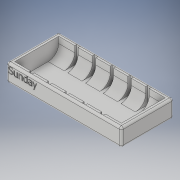
# Autodesk Inventor part: Sunday
Saved by Autodesk Inventor 2019.4 (Build 234330000, 330)
## iProperties
Created: 2020-10-20
Part Number: Sunday
Material: Generic
Document SubType Name: Modeling
Designer: daanswinters
Density: 1 g/cm^3
Appearance: Default
Author: daanswinters
Autodesk Inventor part; units mm, degrees
ref_plane "YZ Plane" through (0, 0, 0) normal (1, 0, 0) x (0, 1, 0)
ref_plane "XZ Plane" through (0, 0, 0) normal (0, 1, 0) x (-1, 0, 0)
ref_plane "XY Plane" through (0, 0, 0) normal (0, 0, 1) x (1, 0, 0)
sketch "Sketch1" plane through (0, 0, 0) normal (0, 0, 1) x (1, 0, 0)
  line L0 (55, -8.5) -> (-55, -8.5)
  line L1 (-55, -8.5) -> (-55, 8.5)
  line L2 (-55, 8.5) -> (55, 8.5)
  line L3 (55, 8.5) -> (55, -8.5)
  line L4 (55, -8.5) -> (-55, 8.5) construction
  line L5 (-55, -8.5) -> (55, 8.5) construction
  point P0 (0, 0)
  dimension "d0" = 110
  dimension "d1" = 17
  constraints: 12 end point, 2 midpoint, 2 parallel, 1 horizontal, 1 perpendicular
  measures "d0" distance of L1.end L2.end
  measures "d1" distance of L0.end L1.end
extrude "Extrusion1" add sketch "Sketch1" along normal blind 50
sketch "Sketch2" plane through (-55, 8.5, 0) normal (0, 1, 0) x (1, 0, 0)
  line L0 (0, 0) -> (0, -50) projected
  line L1 (110, -50) -> (0, -50)
  line L2 (0, -50) -> (0, 0)
  line L3 (0, 0) -> (110, 0)
  line L4 (110, 0) -> (110, -50)
  line L5 (110, -50) -> (0, 0) construction
  line L6 (0, -50) -> (110, 0) construction
  line L7 (106, -46) -> (106, -4)
  line L8 (4, -4) -> (4, -46)
  line L9 (56.15, -2) -> (53.85, -2)
  line L10 (53.85, -48) -> (56.15, -48)
  line L11 (56.15, -2) -> (53.85, -48) construction
  line L12 (53.85, -2) -> (56.15, -48) construction
  line L13 (73.15, -2) -> (70.85, -2)
  line L14 (70.85, -48) -> (73.15, -48)
  line L15 (73.15, -2) -> (70.85, -48) construction
  line L16 (70.85, -2) -> (73.15, -48) construction
  line L17 (0, -25) -> (110, -25) construction
  line L18 (87.85, -2) -> (90.15, -2)
  line L19 (90.15, -48) -> (87.85, -48)
  line L20 (87.85, -2) -> (90.15, -48) construction
  line L21 (90.15, -2) -> (87.85, -48) construction
  line L22 (36.85, -2) -> (39.15, -2)
  line L23 (39.15, -48) -> (36.85, -48)
  line L24 (36.85, -2) -> (39.15, -48) construction
  line L25 (39.15, -2) -> (36.85, -48) construction
  line L26 (19.85, -2) -> (22.15, -2)
  line L27 (22.15, -48) -> (19.85, -48)
  line L28 (19.85, -2) -> (22.15, -48) construction
  line L29 (22.15, -2) -> (19.85, -48) construction
  line L30 (90.15, -2) -> (90.15, -4)
  line L31 (90.15, -46) -> (90.15, -48)
  line L32 (87.85, -48) -> (87.85, -46)
  line L33 (87.85, -4) -> (87.85, -2)
  line L34 (73.15, -48) -> (73.15, -46)
  line L35 (73.15, -4) -> (73.15, -2)
  line L36 (70.85, -2) -> (70.85, -4)
  line L37 (70.85, -46) -> (70.85, -48)
  line L38 (56.15, -4) -> (56.15, -2)
  line L39 (53.85, -2) -> (53.85, -4)
  line L40 (53.85, -46) -> (53.85, -48)
  line L41 (56.15, -48) -> (56.15, -46)
  line L42 (39.15, -2) -> (39.15, -4)
  line L43 (39.15, -46) -> (39.15, -48)
  line L44 (36.85, -48) -> (36.85, -46)
  line L45 (36.85, -4) -> (36.85, -2)
  line L46 (22.15, -2) -> (22.15, -4)
  line L47 (19.85, -48) -> (19.85, -46)
  line L48 (19.85, -4) -> (19.85, -2)
  line L49 (22.15, -46) -> (22.15, -48)
  line L50 (4, -46) -> (19.95, -46)
  line L51 (22.05, -46) -> (36.95, -46)
  line L52 (39.05, -46) -> (53.95, -46)
  line L53 (56.05, -46) -> (70.95, -46)
  line L54 (73.05, -46) -> (87.95, -46)
  line L55 (90.05, -46) -> (106, -46)
  line L56 (106, -4) -> (90.05, -4)
  line L57 (87.95, -4) -> (73.05, -4)
  line L58 (70.95, -4) -> (56.05, -4)
  line L59 (53.95, -4) -> (39.05, -4)
  line L60 (36.95, -4) -> (22.05, -4)
  line L61 (19.95, -4) -> (4, -4)
  point P0 (55, 0)
  point P1 (55, -25)
  point P2 (72, -25)
  point P3 (89, -25)
  point P4 (38, -25)
  point P5 (21, -25)
  dimension "d4" = 65.556
  dimension "d5" = 110
  dimension "d7" = 2.3
  dimension "d8" = 46
  dimension "d9" = 2.3
  dimension "d10" = 46
  dimension "d11" = 0
  dimension "d12" = 2.3
  dimension "d13" = 46
  dimension "d14" = 2.3
  dimension "d15" = 46
  dimension "d16" = 2.3
  dimension "d17" = 46
  dimension "d18" = 17
  dimension "d19" = 17
  dimension "d20" = 17
  dimension "d21" = 17
  dimension "d22" = 2.862
  dimension "d23" = 2.862
  dimension "d24" = 106
  dimension "d25" = 4
  dimension "d26" = 42
  dimension "d27" = 2
  dimension "d28" = 0
  dimension "d29" = 42
  dimension "d30" = 0
  dimension "d31" = 42
  dimension "d32" = 0
  dimension "d33" = 42
  dimension "d34" = 0
  dimension "d35" = 42
  dimension "d36" = 0
  dimension "d37" = 42
  constraints: 122 end point, 73 parallel, 43 point on line, 17 perpendicular, 14 midpoint, 6 horizontal
  measures "d4" angle of L5 L0
  measures "d5" distance between parallel lines of L4 L0
  measures "d7" distance of L10.end L10.start
  measures "d8" distance of L10.start L9.end
  measures "d9" distance of L14.end L14.start
  measures "d10" distance of L14.start L13.end
  measures "d11" distance from line of L17 point (72, -25)
  measures "d12" distance of L19.start L19.end
  measures "d13" distance of L18.end L19.start
  measures "d14" distance of L23.start L23.end
  measures "d15" distance of L22.end L23.start
  measures "d16" distance of L27.start L27.end
  measures "d17" distance of L26.end L27.start
  measures "d18" distance of point (72, -25) point (55, -25)
  measures "d19" distance of point (89, -25) point (72, -25)
  measures "d20" distance of point (38, -25) point (55, -25)
  measures "d21" distance of point (21, -25) point (38, -25)
  measures "d22" angle of L0 L20
  measures "d23" angle of L0 L21
  measures "d24" distance between parallel lines of L7 L0
  measures "d25" distance between parallel lines of L8 L0
  measures "d26" distance between parallel lines of L56 L55
  measures "d27" distance between parallel lines of L56 L18
  measures "d28" distance between parallel lines of L56 L57
  measures "d29" distance between parallel lines of L56 L54
  measures "d30" distance between parallel lines of L56 L58
  measures "d31" distance between parallel lines of L56 L53
  measures "d32" distance between parallel lines of L56 L59
  measures "d33" distance between parallel lines of L56 L52
  measures "d34" distance between parallel lines of L56 L60
  measures "d35" distance between parallel lines of L56 L51
  measures "d36" distance between parallel lines of L56 L61
  measures "d37" distance between parallel lines of L56 L50
extrude "Extrusion2" cut sketch "Sketch2" against normal blind 16 contours L55 L31 L19 L32 L54 L34 L14 L37 L53 L41 L10 L40 L52 L43 L23 L44 L51 L49 L27 L47 L50 L8 L61 L48 L26 L46 L60 L45 L22 L42 L59 L39 L9 L38 L58 L36 L13 L35 L57 L33 L18 L30 L56 L7
fillet "Fillet1" radius 2 12 edges at (-55, 0, 50) (-55, 0, 0) (55, 0, 50) (55, 0, 0) (0, 8.5, 50) (-55, 8.5, 25) (0, 8.5, 0) (55, 8.5, 25) (55, -8.5, 25) (0, -8.5, 50) (-55, -8.5, 25) (0, -8.5, 0)
fillet "Fillet2" radius 10 6 edges at (-43.075, -7.5, 4) (-25.5, -7.5, 4) (-8.5, -7.5, 4) (8.5, -7.5, 4) (25.5, -7.5, 4) (43.075, -7.5, 4)
sketch "Sketch3" plane through (35.15, 8.5, 4) normal (0, 1, 0) x (1, 0, 0)
  line L0 (-70.3, -44) -> (-70.3, -42) projected
  line L1 (-51, 2) -> (-53.3, 2)
  line L2 (-34, 2) -> (-34, 0) projected
  line L3 (-36.3, -44) -> (-36.3, -42) projected
  line L4 (-19.3, -44) -> (-19.3, -42) projected
  line L5 (-2.3, -44) -> (-2.3, -42) projected
  line L6 (0, 2) -> (0, 0) projected
  line L7 (-19.8, 2) -> (-16.5, 2)
  line L8 (-16.5, 2) -> (-16.5, -44)
  line L9 (-16.5, -44) -> (-19.8, -44)
  line L10 (-19.8, -44) -> (-19.8, 2)
  line L11 (-19.8, 2) -> (-16.5, -44) construction
  line L12 (-16.5, 2) -> (-19.8, -44) construction
  line L13 (-2.8, -44) -> (0.5, -44)
  line L14 (0.5, -44) -> (0.5, 2)
  line L15 (0.5, 2) -> (-2.8, 2)
  line L16 (-2.8, 2) -> (-2.8, -44)
  line L17 (-2.8, -44) -> (0.5, 2) construction
  line L18 (0.5, -44) -> (-2.8, 2) construction
  line L19 (-36.8, -44) -> (-33.5, -44)
  line L20 (-33.5, -44) -> (-33.5, 2)
  line L21 (-33.5, 2) -> (-36.8, 2)
  line L22 (-36.8, 2) -> (-36.8, -44)
  line L23 (-36.8, -44) -> (-33.5, 2) construction
  line L24 (-33.5, -44) -> (-36.8, 2) construction
  line L25 (-51, 2) -> (-36.3, 2) projected
  line L26 (-53.8, -44) -> (-50.5, -44)
  line L27 (-50.5, -44) -> (-50.5, 2)
  line L28 (-50.5, 2) -> (-53.8, 2)
  line L29 (-53.8, 2) -> (-53.8, -44)
  line L30 (-53.8, -44) -> (-50.5, 2) construction
  line L31 (-50.5, -44) -> (-53.8, 2) construction
  line L32 (-53.3, -44) -> (-68, -44) projected
  line L33 (-70.8, 2) -> (-67.5, 2)
  line L34 (-67.5, 2) -> (-67.5, -44)
  line L35 (-67.5, -44) -> (-70.8, -44)
  line L36 (-70.8, -44) -> (-70.8, 2)
  line L37 (-70.8, 2) -> (-67.5, -44) construction
  line L38 (-67.5, 2) -> (-70.8, -44) construction
  point P0 (-35.15, 4)
  point P1 (-68, 2)
  point P2 (-17, 2)
  point P3 (-18.15, -21)
  point P4 (-1.15, -21)
  point P5 (-35.15, -21)
  point P6 (-52.15, -21)
  point P7 (-69.15, -21)
  dimension "d42" = 3.3
  dimension "d43" = 46
  dimension "d44" = 3.3
  dimension "d45" = 3.3
  dimension "d46" = 3.3
  dimension "d47" = 3.3
  dimension "d48" = 90
  dimension "d49" = 0.5
  dimension "d50" = 16.5
  dimension "d51" = 33.5
  dimension "d52" = 50.5
  dimension "d53" = 67.5
  dimension "d54" = 46
  dimension "d55" = 0
  dimension "d56" = 53.3
  constraints: 62 end point, 14 parallel, 10 midpoint, 5 horizontal, 5 perpendicular, 3 point on line
  measures "d42" distance of L8.end L9.end
  measures "d43" distance of L7.end L8.end
  measures "d44" distance of L15.end L14.end
  measures "d45" distance of L21.end L20.end
  measures "d46" distance of L28.end L27.end
  measures "d47" distance of L34.end L35.end
  measures "d48" angle of L6 L1
  measures "d49" distance between parallel lines of L6 L14
  measures "d50" distance between parallel lines of L6 L8
  measures "d51" distance between parallel lines of L6 L20
  measures "d52" distance between parallel lines of L6 L27
  measures "d53" distance between parallel lines of L6 L34
  measures "d54" distance between parallel lines of L25 L9
  measures "d55" distance between parallel lines of L15 L25
  measures "d56" distance from line of L1.end L6
extrude "Extrusion3" cut sketch "Sketch3" against normal blind 16
sketch "Sketch4" plane through (0, 0, 50) normal (0, 0, 1) x (1, 0, 0)
  line L0 (-52.9749, 6.5012) -> (53.0345, 6.5012) construction
  line L1 (53.0345, 6.5012) -> (53.0345, -6.5247) construction
  line L2 (53.0345, -6.5247) -> (-52.9749, -6.5247) construction
  line L3 (-52.9749, -6.5247) -> (-52.9749, 6.5012) construction
  spline S0 degree 2 poles (-50.6565, 0.0206) (-51.3189, 0.0206) (-52.2483, 0.2974) (-52.6586, 0.4952) knots 0 0 0 1 2 2 2
  line L4 (-52.6586, 0.4952) -> (-52.6586, 1.5135)
  line L5 (-52.6586, 1.5135) -> (-52.5992, 1.5135)
  spline S1 degree 2 poles (-52.5992, 1.5135) (-52.1988, 1.1378) (-51.1855, 0.7226) (-50.7159, 0.7226) knots 0 0 0 1 2 2 2
  spline S2 degree 2 poles (-50.7159, 0.7226) (-50.0436, 0.7226) (-49.3565, 1.2812) (-49.3565, 1.7409) knots 0 0 0 1 2 2 2
  spline S3 degree 2 poles (-49.3565, 1.7409) (-49.3565, 2.1067) (-49.7173, 2.5615) (-50.1078, 2.6752) knots 0 0 0 1 2 2 2
  spline S4 degree 2 poles (-50.1078, 2.6752) (-50.3896, 2.7542) (-50.8592, 2.863) (-51.2102, 2.952) knots 0 0 0 1 2 2 2
  spline S5 degree 2 poles (-51.2102, 2.952) (-51.5265, 3.036) (-52.0258, 3.2881) (-52.2186, 3.4908) knots 0 0 0 1 2 2 2
  spline S6 degree 2 poles (-52.2186, 3.4908) (-52.4065, 3.6935) (-52.6141, 4.2372) (-52.6141, 4.5931) knots 0 0 0 1 2 2 2
  spline S7 degree 2 poles (-52.6141, 4.5931) (-52.6141, 5.3346) (-51.4573, 6.3381) (-50.5626, 6.3381) knots 0 0 0 1 2 2 2
  spline S8 degree 2 poles (-50.5626, 6.3381) (-50.0485, 6.3381) (-49.1389, 6.1354) (-48.7484, 5.9427) knots 0 0 0 1 2 2 2
  line L6 (-48.7484, 5.9427) -> (-48.7484, 4.9738)
  line L7 (-48.7484, 4.9738) -> (-48.8077, 4.9738)
  spline S9 degree 2 poles (-48.8077, 4.9738) (-49.0994, 5.2407) (-50.009, 5.6362) (-50.5082, 5.6362) knots 0 0 0 1 2 2 2
  spline S10 degree 2 poles (-50.5082, 5.6362) (-51.0718, 5.6362) (-51.7688, 5.1072) (-51.7688, 4.6772) knots 0 0 0 1 2 2 2
  spline S11 degree 2 poles (-51.7688, 4.6772) (-51.7688, 4.2916) (-51.3585, 3.8319) (-50.9729, 3.7281) knots 0 0 0 1 2 2 2
  spline S12 degree 2 poles (-50.9729, 3.7281) (-50.7159, 3.6589) (-49.9694, 3.4809) (-49.7223, 3.4068) knots 0 0 0 1 2 2 2
  spline S13 degree 2 poles (-49.7223, 3.4068) (-49.0945, 3.214) (-48.5112, 2.4379) (-48.5112, 1.8694) knots 0 0 0 1 2 2 2
  spline S14 degree 2 poles (-48.5112, 1.8694) (-48.5112, 1.5085) (-48.8028, 0.8165) (-49.0648, 0.5743) knots 0 0 0 1 2 2 2
  spline S15 degree 2 poles (-49.0648, 0.5743) (-49.3565, 0.3073) (-50.0979, 0.0206) (-50.6565, 0.0206) knots 0 0 0 1 2 2 2
  line L8 (-44.1858, 0.1294) -> (-44.9569, 0.1294)
  line L9 (-44.9569, 0.1294) -> (-44.9569, 0.6336)
  spline S16 degree 2 poles (-44.9569, 0.6336) (-45.3129, 0.3222) (-45.9505, 0.0008) (-46.346, 0.0008) knots 0 0 0 1 2 2 2
  spline S17 degree 2 poles (-46.346, 0.0008) (-46.6426, 0.0008) (-47.1715, 0.1986) (-47.3643, 0.4111) knots 0 0 0 1 2 2 2
  spline S18 degree 2 poles (-47.3643, 0.4111) (-47.562, 0.6237) (-47.7795, 1.2713) (-47.7795, 1.7359) knots 0 0 0 1 2 2 2
  line L10 (-47.7795, 1.7359) -> (-47.7795, 4.7068)
  line L11 (-47.7795, 4.7068) -> (-47.0084, 4.7068)
  line L12 (-47.0084, 4.7068) -> (-47.0084, 2.0968)
  spline S19 degree 2 poles (-47.0084, 2.0968) (-47.0084, 1.731) (-46.954, 1.2515) (-46.8601, 1.0735) knots 0 0 0 1 2 2 2
  spline S20 degree 2 poles (-46.8601, 1.0735) (-46.7662, 0.8956) (-46.4449, 0.7324) (-46.1433, 0.7324) knots 0 0 0 1 2 2 2
  spline S21 degree 2 poles (-46.1433, 0.7324) (-45.8616, 0.7324) (-45.2239, 1.0538) (-44.9569, 1.2861) knots 0 0 0 1 2 2 2
  line L13 (-44.9569, 1.2861) -> (-44.9569, 4.7068)
  line L14 (-44.9569, 4.7068) -> (-44.1858, 4.7068)
  line L15 (-44.1858, 4.7068) -> (-44.1858, 0.1294)
  line L16 (-39.4748, 0.1294) -> (-40.246, 0.1294)
  line L17 (-40.246, 0.1294) -> (-40.246, 2.7394)
  spline S22 degree 2 poles (-40.246, 2.7394) (-40.246, 3.0558) (-40.3053, 3.5995) (-40.3943, 3.7627) knots 0 0 0 1 2 2 2
  spline S23 degree 2 poles (-40.3943, 3.7627) (-40.4882, 3.9357) (-40.8244, 4.1038) (-41.1111, 4.1038) knots 0 0 0 1 2 2 2
  spline S24 degree 2 poles (-41.1111, 4.1038) (-41.3978, 4.1038) (-42.0058, 3.7973) (-42.2975, 3.5501) knots 0 0 0 1 2 2 2
  line L18 (-42.2975, 3.5501) -> (-42.2975, 0.1294)
  line L19 (-42.2975, 0.1294) -> (-43.0686, 0.1294)
  line L20 (-43.0686, 0.1294) -> (-43.0686, 4.7068)
  line L21 (-43.0686, 4.7068) -> (-42.2975, 4.7068)
  line L22 (-42.2975, 4.7068) -> (-42.2975, 4.1977)
  spline S25 degree 2 poles (-42.2975, 4.1977) (-41.9514, 4.5091) (-41.2841, 4.8354) (-40.9084, 4.8354) knots 0 0 0 1 2 2 2
  spline S26 degree 2 poles (-40.9084, 4.8354) (-40.2361, 4.8354) (-39.4748, 3.9456) (-39.4748, 3.1003) knots 0 0 0 1 2 2 2
  line L23 (-39.4748, 3.1003) -> (-39.4748, 0.1294)
  line L24 (-34.8727, 0.1294) -> (-35.6438, 0.1294)
  line L25 (-35.6438, 0.1294) -> (-35.6438, 0.594)
  spline S27 degree 2 poles (-35.6438, 0.594) (-35.8218, 0.4457) (-36.0838, 0.248) (-36.2617, 0.164) knots 0 0 0 1 2 2 2
  spline S28 degree 2 poles (-36.2617, 0.164) (-36.4248, 0.0849) (-36.7758, 0.0008) (-37.0082, 0.0008) knots 0 0 0 1 2 2 2
  spline S29 degree 2 poles (-37.0082, 0.0008) (-37.3838, 0.0008) (-38.0166, 0.3123) (-38.239, 0.6138) knots 0 0 0 1 2 2 2
  spline S30 degree 2 poles (-38.239, 0.6138) (-38.4615, 0.9153) (-38.7086, 1.8051) (-38.7086, 2.3835) knots 0 0 0 1 2 2 2
  spline S31 degree 2 poles (-38.7086, 2.3835) (-38.7086, 2.9866) (-38.3972, 3.8665) (-38.1253, 4.1977) knots 0 0 0 1 2 2 2
  spline S32 degree 2 poles (-38.1253, 4.1977) (-37.8732, 4.4943) (-37.1663, 4.8354) (-36.7758, 4.8354) knots 0 0 0 1 2 2 2
  spline S33 degree 2 poles (-36.7758, 4.8354) (-36.4347, 4.8354) (-35.9256, 4.6821) (-35.6438, 4.5239) knots 0 0 0 1 2 2 2
  line L26 (-35.6438, 4.5239) -> (-35.6438, 6.5012)
  line L27 (-35.6438, 6.5012) -> (-34.8727, 6.5012)
  line L28 (-34.8727, 6.5012) -> (-34.8727, 0.1294)
  line L29 (-35.6438, 1.2416) -> (-35.6438, 3.8863)
  spline S34 degree 2 poles (-35.6438, 3.8863) (-35.9305, 4.0247) (-36.3853, 4.1285) (-36.6473, 4.1285) knots 0 0 0 1 2 2 2
  spline S35 degree 2 poles (-36.6473, 4.1285) (-37.2405, 4.1285) (-37.9128, 3.2387) (-37.9128, 2.3983) knots 0 0 0 1 2 2 2
  spline S36 degree 2 poles (-37.9128, 2.3983) (-37.9128, 1.5876) (-37.3987, 0.7324) (-36.8302, 0.7324) knots 0 0 0 1 2 2 2
  spline S37 degree 2 poles (-36.8302, 0.7324) (-36.5287, 0.7324) (-35.9157, 1.0093) (-35.6438, 1.2416) knots 0 0 0 1 2 2 2
  spline S38 degree 2 poles (-31.2047, 0.6138) (-31.2987, 0.5446) (-31.615, 0.2974) (-31.7633, 0.2233) knots 0 0 0 1 2 2 2
  spline S39 degree 2 poles (-31.7633, 0.2233) (-31.966, 0.1145) (-32.3466, 0.0008) (-32.6927, 0.0008) knots 0 0 0 1 2 2 2
  spline S40 degree 2 poles (-32.6927, 0.0008) (-32.9744, 0.0008) (-33.4836, 0.2134) (-33.6764, 0.4062) knots 0 0 0 1 2 2 2
  spline S41 degree 2 poles (-33.6764, 0.4062) (-33.8593, 0.594) (-34.0817, 1.1477) (-34.0817, 1.4542) knots 0 0 0 1 2 2 2
  spline S42 degree 2 poles (-34.0817, 1.4542) (-34.0817, 1.9287) (-33.6813, 2.601) (-33.2463, 2.7938) knots 0 0 0 1 2 2 2
  spline S43 degree 2 poles (-33.2463, 2.7938) (-32.8607, 2.9718) (-31.8128, 3.1052) (-31.2047, 3.1398) knots 0 0 0 1 2 2 2
  line L30 (-31.2047, 3.1398) -> (-31.2047, 3.2881)
  spline S44 degree 2 poles (-31.2047, 3.2881) (-31.2047, 3.5551) (-31.3679, 3.8863) (-31.5162, 3.9802) knots 0 0 0 1 2 2 2
  spline S45 degree 2 poles (-31.5162, 3.9802) (-31.6645, 4.0741) (-32.0896, 4.1334) (-32.317, 4.1334) knots 0 0 0 1 2 2 2
  spline S46 degree 2 poles (-32.317, 4.1334) (-32.5839, 4.1334) (-33.3056, 3.9752) (-33.6665, 3.822) knots 0 0 0 1 2 2 2
  line L31 (-33.6665, 3.822) -> (-33.711, 3.822)
  line L32 (-33.711, 3.822) -> (-33.711, 4.608)
  spline S47 degree 2 poles (-33.711, 4.608) (-33.4984, 4.6673) (-32.7026, 4.8156) (-32.312, 4.8156) knots 0 0 0 1 2 2 2
  spline S48 degree 2 poles (-32.312, 4.8156) (-31.8375, 4.8156) (-31.1899, 4.6673) (-30.9329, 4.4745) knots 0 0 0 1 2 2 2
  spline S49 degree 2 poles (-30.9329, 4.4745) (-30.6808, 4.2867) (-30.4336, 3.6885) (-30.4336, 3.2585) knots 0 0 0 1 2 2 2
  line L33 (-30.4336, 3.2585) -> (-30.4336, 0.1294)
  line L34 (-30.4336, 0.1294) -> (-31.2047, 0.1294)
  line L35 (-31.2047, 0.1294) -> (-31.2047, 0.6138)
  line L36 (-31.2047, 1.2564) -> (-31.2047, 2.5269)
  spline S50 degree 2 poles (-31.2047, 2.5269) (-31.4816, 2.5021) (-32.317, 2.4181) (-32.579, 2.339) knots 0 0 0 1 2 2 2
  spline S51 degree 2 poles (-32.579, 2.339) (-32.8855, 2.2451) (-33.2859, 1.8546) (-33.2859, 1.5085) knots 0 0 0 1 2 2 2
  spline S52 degree 2 poles (-33.2859, 1.5085) (-33.2859, 1.1131) (-32.841, 0.7127) (-32.4159, 0.7127) knots 0 0 0 1 2 2 2
  spline S53 degree 2 poles (-32.4159, 0.7127) (-32.055, 0.7127) (-31.4618, 1.0241) (-31.2047, 1.2564) knots 0 0 0 1 2 2 2
  line L37 (-25.7573, 4.7068) -> (-28.219, -1.5563)
  line L38 (-28.219, -1.5563) -> (-29.0445, -1.5563)
  line L39 (-29.0445, -1.5563) -> (-28.224, 0.3518)
  line L40 (-28.224, 0.3518) -> (-29.8849, 4.7068)
  line L41 (-29.8849, 4.7068) -> (-29.0544, 4.7068)
  line L42 (-29.0544, 4.7068) -> (-27.8038, 1.3158)
  line L43 (-27.8038, 1.3158) -> (-26.5581, 4.7068)
  line L44 (-26.5581, 4.7068) -> (-25.7573, 4.7068)
  point P0 (0, 0)
  constraints: 2 other
extrude "Extrusion4" cut sketch "Sketch4" against normal blind 0.5
fillet "Fillet3" radius 10 6 edges at (-43.325, -7.5, 46) (-25.5, -7.5, 46) (-8.5, -7.5, 46) (8.5, -7.5, 46) (25.5, -7.5, 46) (43.325, -7.5, 46)
body "Solid1"
